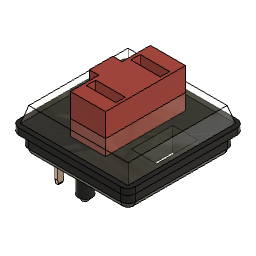
kailh choc switch (wrongly cadded pins) v1 (Autodesk Fusion 360 design; units mm, degrees)
Autodesk Fusion 360 part; units mm, degrees
note: some values were not read from the file. Set by a fixed rule: which sketch regions a step uses.
sketch "Sketch1" plane through (0, 0, 0) normal (0, 0, 1) x (1, 0, 0)
  circle A0 centre (0, 0) radius 1.6
  line L0 (6.9, 6.9) -> (-6.9, 6.9)
  line L1 (-6.9, 6.9) -> (-6.9, -6.9)
  line L2 (-6.9, -6.9) -> (6.9, -6.9)
  line L3 (6.9, -6.9) -> (6.9, 6.9)
  line L4 (6.9, 6.9) -> (-6.9, -6.9) construction
  line L5 (-6.9, 6.9) -> (6.9, -6.9) construction
  circle A1 centre (0, 5.5) radius 0.9
  circle A2 centre (0, -5.5) radius 0.9
  line L6 (-6.9, 0) -> (6.9, 0) construction
  line L7 (0, -6.9) -> (0, 6.9) construction
  line L8 (6.325, 2.65) -> (3.075, 2.65)
  line L9 (3.075, 2.65) -> (3.075, -2.65)
  line L10 (3.075, -2.65) -> (6.325, -2.65)
  line L11 (6.325, -2.65) -> (6.325, 2.65)
  line L12 (6.325, 2.65) -> (3.075, -2.65) construction
  line L13 (3.075, 2.65) -> (6.325, -2.65) construction
  line L14 (-5.75, 0.45) -> (-6.05, 0.45)
  line L15 (-6.05, 0.45) -> (-6.05, -0.45)
  line L16 (-6.05, -0.45) -> (-5.75, -0.45)
  line L17 (-5.75, -0.45) -> (-5.75, 0.45)
  line L18 (-5.75, 0.45) -> (-6.05, -0.45) construction
  line L19 (-6.05, 0.45) -> (-5.75, -0.45) construction
  line L20 (-3.625, -4.6) -> (-3.975, -4.6)
  line L21 (-3.975, -4.6) -> (-3.975, -5.4)
  line L22 (-3.975, -5.4) -> (-3.625, -5.4)
  line L23 (-3.625, -5.4) -> (-3.625, -4.6)
  line L24 (-3.625, -4.6) -> (-3.975, -5.4) construction
  line L25 (-3.975, -4.6) -> (-3.625, -5.4) construction
  line L26 (-7.5, -7.5) -> (7.5, -7.5)
  line L27 (7.5, -7.5) -> (7.5, 7.5)
  line L28 (7.5, 7.5) -> (-7.5, 7.5)
  line L29 (-7.5, 7.5) -> (-7.5, -7.5)
  point P0 (4.7, 0)
  point P1 (-5.9, 0)
  point P2 (-3.8, -5)
  dimension "d1" = 3.2
  dimension "d2" = 13.8
  dimension "d3" = 13.8
  dimension "d4" = 1.8
  dimension "d5" = 1.8
  dimension "d6" = 11
  dimension "d7" = 0.6
  dimension "d35" = 5.3
  dimension "d36" = 3.25
  dimension "d37" = 4.7
  dimension "d38" = 0.9
  dimension "d39" = 0.3
  dimension "d40" = 5.9
  dimension "d41" = 0.8
  dimension "d42" = 0.35
  dimension "d43" = 5
  dimension "d45" = 3.8
  constraint coincident A0.centre origin
  constraint perpendicular L0 L1
  constraint parallel L0 L2
  constraint parallel L1 L3
  constraint horizontal L0
  constraint coincident L4 A0.centre
  constraint coincident L5 A0.centre
  constraint midpoint L1 L6.start
  constraint midpoint L3 L6.end
  constraint midpoint L2 L7.start
  constraint midpoint L0 L7.end
  constraint coincident A1.centre L7
  constraint coincident A2.centre L7
  constraint symmetric A1.centre A2.centre L6
  constraint perpendicular L8 L9
  constraint parallel L8 L10
  constraint parallel L9 L11
  constraint horizontal L8
  constraint coincident L12 P0
  constraint coincident L13 P0
  constraint coincident L6 P0
  constraint perpendicular L14 L15
  constraint parallel L14 L16
  constraint parallel L15 L17
  constraint horizontal L14
  constraint coincident L18 P1
  constraint coincident L19 P1
  constraint coincident L6 P1
  constraint perpendicular L20 L21
  constraint parallel L20 L22
  constraint parallel L21 L23
  constraint horizontal L20
  constraint coincident L24 P2
  constraint coincident L25 P2
  measures "d1" diameter of A0
  measures "d2" distance of L1.end L2.end
  measures "d3" distance of L0.end L1.end
  measures "d4" diameter of A1
  measures "d5" diameter of A2
  measures "d6" vertical distance of A1.centre A2.centre
  measures "d35" distance of L8.end L9.end
  measures "d36" distance of L9.end L10.end
  measures "d37" horizontal distance of A0.centre P0
  measures "d38" distance of L14.end L15.end
  measures "d39" distance of L15.end L16.end
  measures "d40" horizontal distance of A0.centre P1
  measures "d41" distance of L20.end L21.end
  measures "d42" distance of L21.end L22.end
  measures "d43" distance of L6 P2
  measures "d45" distance of L7 P2
extrude "Extrude1" add sketch "Sketch1" against normal blind 3 contours A0 | L0 L1 L2 L3 | A1 | A2 | L14 L15 L16 L17 | L20 L21 L22 L23 makes body 1
extrude "Extrude2" add sketch "Sketch1" against normal blind 0.8 contours L26 L27 L28 L29 bodies 1
extrude "Extrude3" add sketch "Sketch1" against normal blind 2.65 from surface at -3 contours A0 | A1 | A2 bodies 1
fillet "Fillet1" radius 1 8 edges at (6.9, -6.9, -1.9) (7.5, -7.5, -0.4) (7.5, 7.5, -0.4) (6.9, 6.9, -1.9) (-7.5, -7.5, -0.4) (-6.9, -6.9, -1.9) (-6.9, 6.9, -1.9) (-7.5, 7.5, -0.4) on bodies 1
chamfer "Chamfer1" distance 0.7 angle 30 8 edges at (6.6071, -6.6071, -3) (6.9, 0, -3) (6.6071, 6.6071, -3) (0, 6.9, -3) (-6.6071, 6.6071, -3) (-6.9, 0, -3) (-6.6071, -6.6071, -3) (0, -6.9, -3) measured on face at (5.9476, -6.8989, -1.5333) measured on face at (-5.1333, 0, -3) measured on face at (5.9476, 6.8989, -1.5333) measured on face at (-5.1333, 0, -3) measured on face at (-6.5182, 6.6861, -1.5333) measured on face at (-5.1333, 0, -3) measured on face at (-6.8989, -5.9476, -1.5333) measured on face at (-5.1333, 0, -3) on bodies 1
chamfer "Chamfer2" distance 0.5 angle 50 3 edges at (-0.8391, 5.8255, -5.65) (-1.4917, 0.5786, -5.65) (-0.8391, -5.1745, -5.65) measured on face at (-0.0239, 5.7793, -5.65) measured on face at (0.5957, -0.3358, -5.65) measured on face at (0.0239, -5.7793, -5.65) on bodies 1
extrude "Extrude4" add sketch "Sketch1" along normal blind 2 draft -15 separate body contours A0 | L0 L1 L2 L3 | A1 | A2 | L8 L9 L10 L11 | L14 L15 L16 L17 | L20 L21 L22 L23 makes body 2
sketch "Sketch2" plane through (0, 0, 2) normal (0, 0, 1) x (1, 0, 0)
  line L0 (6.3641, 6.3641) -> (-6.3641, 6.3641)
  line L1 (6.3641, -6.3641) -> (6.3641, 6.3641)
  line L2 (-6.3641, -6.3641) -> (6.3641, -6.3641)
  line L3 (-6.3641, 6.3641) -> (-6.3641, -6.3641)
  line L4 (2.25, 5.125) -> (-2.25, 5.125)
  line L5 (-2.25, 5.125) -> (-2.25, -5.125)
  line L6 (-2.25, -5.125) -> (2.25, -5.125)
  line L7 (2.25, -5.125) -> (2.25, 5.125)
  line L8 (2.25, 5.125) -> (-2.25, -5.125) construction
  line L9 (-2.25, 5.125) -> (2.25, -5.125) construction
  line L10 (1.9, 2.25) -> (-1.9, 2.25)
  line L11 (-1.9, 2.25) -> (-1.9, 3.45)
  line L12 (-1.9, 3.45) -> (1.9, 3.45)
  line L13 (1.9, 3.45) -> (1.9, 2.25)
  line L14 (1.9, 2.25) -> (-1.9, 3.45) construction
  line L15 (-1.9, 2.25) -> (1.9, 3.45) construction
  line L16 (1.9, -3.45) -> (-1.9, -3.45)
  line L17 (-1.9, -3.45) -> (-1.9, -2.25)
  line L18 (-1.9, -2.25) -> (1.9, -2.25)
  line L19 (1.9, -2.25) -> (1.9, -3.45)
  line L20 (1.9, -3.45) -> (-1.9, -2.25) construction
  line L21 (-1.9, -3.45) -> (1.9, -2.25) construction
  line L22 (-6.3641, 0) -> (6.3641, 0) construction
  line L23 (0, 6.3641) -> (0, -6.3641) construction
  line L24 (-3.45, 1.5) -> (-2.25, 1.5)
  line L25 (-2.25, 1.5) -> (-2.25, -1.5)
  line L26 (-2.25, -1.5) -> (-3.45, -1.5)
  line L27 (-3.45, -1.5) -> (-3.45, 1.5)
  point P0 (0, 2.85)
  point P1 (0, -2.85)
  dimension "d22" = 3.8
  dimension "d23" = 1.2
  dimension "d24" = 3.8
  dimension "d25" = 1.2
  dimension "d26" = 4.5
  dimension "d27" = 10.25
  dimension "d28" = 5.7
  dimension "d29" = 1.2
  dimension "d30" = 3
  constraint perpendicular L4 L5
  constraint parallel L4 L6
  constraint parallel L5 L7
  constraint horizontal L4
  constraint coincident L8 origin
  constraint coincident L9 origin
  constraint perpendicular L10 L11
  constraint parallel L10 L12
  constraint parallel L11 L13
  constraint horizontal L10
  constraint coincident L14 P0
  constraint coincident L15 P0
  constraint perpendicular L16 L17
  constraint parallel L16 L18
  constraint parallel L17 L19
  constraint horizontal L16
  constraint coincident L20 P1
  constraint coincident L21 P1
  constraint midpoint L3 L22.start
  constraint midpoint L1 L22.end
  constraint symmetric P0 P1 L22
  constraint midpoint L0 L23.start
  constraint midpoint L2 L23.end
  constraint coincident P0 L23
  constraint horizontal L24
  constraint vertical L25
  constraint horizontal L26
  constraint vertical L27
  constraint coincident L5 L24.end
  constraint midpoint L5 L25
  measures "d22" distance of L11.end L12.end
  measures "d23" distance of L10.end L11.end
  measures "d24" distance of L17.end L18.end
  measures "d25" distance of L16.end L17.end
  measures "d26" horizontal distance of L4.start L4.end
  measures "d27" vertical distance of L4.start L6.end
  measures "d28" vertical distance of P0 P1
  measures "d29" horizontal distance of L24.start L24.end
  measures "d30" distance of L24 L26
extrude "Extrude5" add sketch "Sketch2" against normal blind 2 separate body contours L4 L5 L6 L7 L25 | L5 L24 L25 L26 L27 | L10 L11 L12 L13 | L16 L17 L18 L19 makes body 3
extrude "Extrude6" add sketch "Sketch2" along normal blind 3 contours L4 L5 L6 L7 L25 | L5 L24 L25 L26 L27 bodies 3
combine "Combine1" operation cut target body 2 tool bodies 3 keep tools
extrude "Extrude7" add sketch "Sketch1" against normal blind 3 from surface at -3 separate body contours L14 L15 L16 L17 | L20 L21 L22 L23 makes body 4 at (-3.625, -5.1333, -4) makes body 5 at (-5.75, -0.15, -4)
chamfer "Chamfer3" distance 0.05 angle 70 4 edges at (-3.625, -5, -6) (-3.975, -5, -6) (-5.75, 0, -6) (-6.05, 0, -6) measured on face at (-3.7417, -5.1333, -6) measured on face at (-3.7417, -5.1333, -6) measured on face at (-5.85, -0.15, -6) measured on face at (-5.85, -0.15, -6) on bodies 4 5
chamfer "Chamfer4" distance 0.1 angle 80 4 edges at (-3.8, -5.4, -6) (-3.8, -4.6, -6) (-5.9, -0.45, -6) (-5.9, 0.45, -6) measured on face at (-3.7583, -5.1333, -6) measured on face at (-3.7583, -5.1333, -6) measured on face at (-5.8667, -0.15, -6) measured on face at (-5.8667, -0.15, -6) on bodies 4 5
combine "Combine2" operation cut target body 1 tool bodies 2 keep tools
named bodies: "Base", "Top", "Stem"
